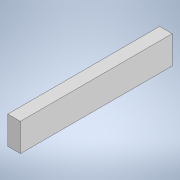
# Autodesk Inventor part: 2x4GarageMountPoint
Saved by Autodesk Inventor 2022.1 (Build 261234020, 234B)
## iProperties
Created: 2021-10-20
Part Number: 2x4GarageMountPoint
Material: Generic
Document SubType Name: Modeling
Designer: robst
Density: 1 g/cm^3
Appearance: Default
Author: robst
Autodesk Inventor part; units mm, degrees
ref_plane "YZ Plane" through (0, 0, 0) normal (1, 0, 0) x (0, 1, 0)
ref_plane "XZ Plane" through (0, 0, 0) normal (0, 1, 0) x (-1, 0, 0)
ref_plane "XY Plane" through (0, 0, 0) normal (0, 0, 1) x (1, 0, 0)
sketch "Sketch1" plane through (0, 0, 0) normal (0, 0, 1) x (1, 0, 0)
  line L0 (-19.05, -42.1005) -> (19.05, -42.1005)
  line L1 (19.05, -42.1005) -> (19.05, 42.1005)
  line L2 (19.05, 42.1005) -> (-19.05, 42.1005)
  line L3 (-19.05, 42.1005) -> (-19.05, -42.1005)
  line L4 (-19.05, -42.1005) -> (19.05, 42.1005) construction
  line L5 (19.05, -42.1005) -> (-19.05, 42.1005) construction
  point P0 (0, 0)
  dimension "d0" = 84.201
  dimension "d1" = 38.1
  constraints: 12 end point, 2 midpoint, 2 parallel, 1 horizontal, 1 perpendicular
  measures "d0" distance of L2.end L0.start
  measures "d1" distance of L1.end L2.end
extrude "Extrusion1" add sketch "Sketch1" along normal mid plane 457.2
equation "\"d0\" = depth"
equation "\"d1\" = width"
equation "\"d2\" = length"
equation "\"width\" = 38.1"
equation "\"depth\" = 84.201"
equation "\"length\" = 457.2"
body "Solid1"
